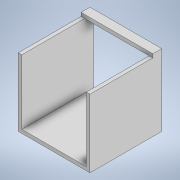
# Autodesk Inventor part: 3SR02_振子支え
Saved by Autodesk Inventor 2021 (Build 250183000, 183)
## iProperties
Created: 2021-04-19
Part Number: 3SR02_振子支え
Material: 一般
Document SubType Name: Modeling
Designer: ryusei
Density: 1 g/cm^3
Appearance: 既定
Author: ryusei
Autodesk Inventor part; units mm, degrees
ref_plane "YZ Plane" through (0, 0, 0) normal (1, 0, 0) x (0, 1, 0)
ref_plane "XZ Plane" through (0, 0, 0) normal (0, 1, 0) x (-1, 0, 0)
ref_plane "XY Plane" through (0, 0, 0) normal (0, 0, 1) x (1, 0, 0)
sketch "スケッチ1" plane through (0, 0, 0) normal (0, 0, 1) x (1, 0, 0)
  line L0 (0, 0) -> (40, 0)
  line L1 (40, 0) -> (40, 40)
  line L2 (40, 40) -> (0, 40)
  line L3 (0, 40) -> (0, 0)
  dimension "d0" = 40
  dimension "d1" = 40
  constraints: 8 end point, 2 parallel, 1 horizontal, 1 perpendicular
  measures "d0" distance between parallel lines of L1 L3
  measures "d1" distance between parallel lines of L0 L2
extrude "押し出し1" add sketch "スケッチ1" along normal blind 40
sketch "スケッチ2" plane through (0, 0, 0) normal (0, 0, -1) x (-1, 0, 0)
  point P0 (0, 0)
sketch "スケッチ3" plane through (0, 0, 40) normal (0, 0, 1) x (1, 0, 0)
  line L0 (2, 2) -> (38, 2)
  line L1 (38, 2) -> (38, 38)
  line L2 (38, 38) -> (2, 38)
  line L3 (2, 38) -> (2, 2)
  line L4 (0, 40) -> (0, 0) projected
  line L5 (40, 40) -> (0, 40) projected
  line L6 (40, 0) -> (40, 40) projected
  line L7 (0, 0) -> (40, 0) projected
  dimension "d4" = 2
  dimension "d5" = 2
  dimension "d6" = 2
  dimension "d7" = 2
  constraints: 8 end point, 2 parallel, 1 horizontal, 1 perpendicular
  measures "d4" distance between parallel lines of L3 L4
  measures "d5" distance between parallel lines of L5 L2
  measures "d6" distance between parallel lines of L6 L1
  measures "d7" distance between parallel lines of L7 L0
extrude "押し出し2" cut sketch "スケッチ3" against normal through all contours L3 L2 L1 L0
sketch "スケッチ4" plane through (0, 40, 0) normal (0, 1, 0) x (1, 0, 0)
  line L0 (0, 0) -> (0, -40) projected
  line L1 (40, 0) -> (40, -40) projected
  line L2 (0, -40) -> (40, -40)
  line L3 (40, -40) -> (40, -5)
  line L4 (40, -5) -> (0, -5)
  line L5 (0, -5) -> (0, -40)
  line L6 (40, 0) -> (0, 0) projected
  point P0 (0, -5)
  dimension "d10" = 5
  constraints: 8 end point, 2 parallel, 1 horizontal, 1 perpendicular, 1 point on line
  measures "d10" distance between parallel lines of L6 L4
extrude "押し出し3" cut sketch "スケッチ4" against normal blind 2 contours L4 L1 L2 L0
